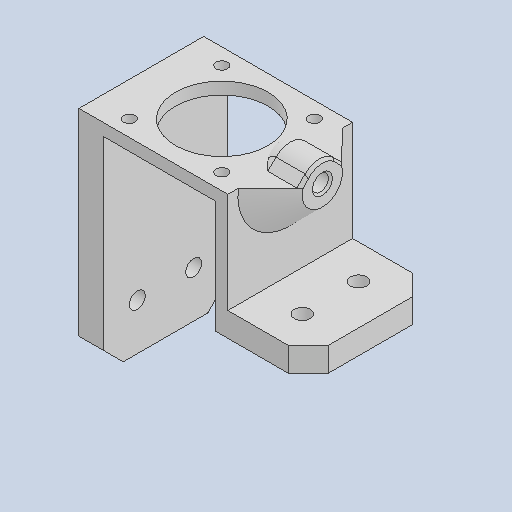
# Autodesk Inventor part: Motor Mount
Saved by Autodesk Inventor 2022 (Build 260153000, 153)
## iProperties
Created: 2022-04-23
Part Number: Motor Mount
Material: Generic
Document SubType Name: Modeling
Designer: Nick
Density: 1 g/cm^3
Appearance: Default
Author: Nick
Autodesk Inventor part; units mm, degrees
ref_plane "YZ Plane" through (0, 0, 0) normal (1, 0, 0) x (0, 1, 0)
ref_plane "XZ Plane" through (0, 0, 0) normal (0, 1, 0) x (-1, 0, 0)
ref_plane "XY Plane" through (0, 0, 0) normal (0, 0, 1) x (1, 0, 0)
sketch "Sketch1" plane through (0, 0, 0) normal (0, 0, 1) x (1, 0, 0)
  line L0 (0, 0) -> (0, 54.05)
  line L1 (0, 54.05) -> (37, 54.05)
  line L2 (37, 54.05) -> (37, 29.05)
  line L3 (37, 29.05) -> (57, 29.05)
  line L4 (57, 29.05) -> (57, 23.05)
  line L5 (57, 23.05) -> (34, 23.05)
  line L6 (34, 23.05) -> (34, 51.05)
  line L7 (34, 51.05) -> (6, 51.05)
  line L8 (6, 51.05) -> (6, 0)
  line L9 (6, 0) -> (0, 0)
  dimension "d0" = 6
  dimension "d1" = 3
  dimension "d2" = 3
  dimension "d3" = 28
  dimension "d5" = 6
  dimension "d6" = 28
  dimension "d7" = 20
  dimension "d60" = 23.05
  constraints: 20 end point, 6 perpendicular, 3 vertical, 1 parallel
  measures "d0" distance of L8.end L0.start
  measures "d1" distance between parallel lines of L1 L7
  measures "d2" distance between parallel lines of L2 L6
  measures "d3" distance of L6.end L7.end
  measures "d5" distance of L3.end L4.end
  measures "d6" distance of L5.end L6.end
  measures "d7" distance of L2.end L3.end
  measures "d60" distance between parallel lines of L9 L5
extrude "Extrusion1" add sketch "Sketch1" along normal blind 31
sketch "Sketch2" plane through (0, 54.05, 0) normal (0, 1, 0) x (1, 0, 0)
  line L0 (8.5, -27) -> (31.5, -27) construction
  line L1 (31.5, -27) -> (31.5, -4) construction
  line L2 (31.5, -4) -> (8.5, -4) construction
  line L3 (8.5, -4) -> (8.5, -27) construction
  line L4 (0, 0) -> (0, -31) construction
  line L5 (37, 0) -> (0, 0) construction
  line L6 (6, 0) -> (34, 0) projected
  line L7 (34, 0) -> (34, -31) projected
  line L8 (6, -31) -> (34, -31) projected
  line L9 (6, 0) -> (6, -31) projected
  point P0 (20, -15.5)
  point P1 (8.5, -15.5)
  point P2 (20, -4)
  point P3 (0, -15.5)
  point P4 (20, 0)
  dimension "d10" = 23
  constraints: 8 end point, 4 midpoint, 2 coincident, 2 horizontal alignment, 2 parallel, 2 perpendicular, 2 vertical alignment, 1 horizontal
  measures "d10" distance of L2.end L0.start
hole "Hole1" at (8.5, 54.05, 27) at (8.5, 54.05, 4) at (31.5, 54.05, 4) at (31.5, 54.05, 27) direction (0, -1, 0) diameter 2.9 end through all
hole "Hole2" at (20, 54.05, 15.5) direction (0, -1, 0) diameter 23 end through all
sketch "Sketch3" plane through (37, 29.05, 0) normal (1, 0, 0) x (0, 0, -1)
  circle A0 centre (-15.5, 23.5) radius 2
  line L0 (0, -6) -> (-31, -6) projected
  circle A1 centre (-15.5, 23.5) radius 5
  point P0 (0, -29.05)
  point P1 (-15.5, -6)
  dimension "d25" = 29.5
  dimension "d26" = 4
  dimension "d27" = 3
  constraints: 2 centre point, 1 midpoint, 1 vertical alignment
  measures "d25" distance from line of A0.centre L0
  measures "d26" diameter of A0
  measures "d27" radial gap between concentric circles of A0 A1
extrude "Extrusion2" add sketch "Sketch3" along normal blind 8
chamfer "Chamfer1" distance 8 angle 45 2 edges at (37, 53.3088, 10.5579) (37, 47.6079, 16.2588)
chamfer "Chamfer2" distance 0.5 angle 45 1 edges at (45, 52.55, 17.5)
sketch "Sketch7" plane through (37, 29.05, 0) normal (0, 1, 0) x (1, 0, 0)
  line L0 (20, 0) -> (0, 0) projected
  line L1 (0, 0) -> (0, -31) projected
  line L2 (20, -31) -> (0, -31) projected
  line L3 (20, 0) -> (20, -31) projected
  point P0 (-37, 0)
  point P1 (10, -22.5)
  point P2 (10, -8.5)
  point P3 (10, -31)
  dimension "d61" = 14
  dimension "d62" = 8.5
  dimension "d63" = 8.5
  constraints: 2 vertical alignment, 1 midpoint
  measures "d61" distance of point (10, -22.5) point (10, -8.5)
  measures "d62" distance of point (10, -31) point (10, -22.5)
  measures "d63" distance from line of L0 point (10, -8.5)
hole "Hole5" at (47, 29.05, 22.5) at (47, 29.05, 8.5) direction (0, -1, 0) diameter 4 end through all
sketch "Sketch8" plane through (0, 0, 0) normal (-1, 0, 0) x (0, 0, 1)
  line L0 (0, 54.05) -> (0, 0) projected
  line L1 (31, 54.05) -> (31, 0) projected
  line L2 (0, 0) -> (31, 0) projected
  line L3 (0, 0) -> (31, 0) construction
  line L4 (31, 0) -> (31, 51.05) construction
  line L5 (0, 0) -> (31, 0) construction
  line L6 (31, 0) -> (31, 23.05) construction
  line L7 (31, 23.05) -> (0, 23.05) construction
  line L8 (0, 23.05) -> (0, 0) construction
  point P0 (8.5, 11.525)
  point P1 (22.5, 11.525)
  point P2 (0, 11.525)
  dimension "d71" = 14
  dimension "d72" = 8.5
  dimension "d73" = 8.5
  dimension "d75" = 23.05
  constraints: 8 end point, 2 horizontal alignment, 2 parallel, 1 horizontal, 1 midpoint, 1 perpendicular, 1 point on line
  measures "d71" distance of point (22.5, 11.525) point (8.5, 11.525)
  measures "d72" distance from line of L0 point (8.5, 11.525)
  measures "d73" distance from line of L1 point (22.5, 11.525)
  measures "d75" distance of L6.end L5.end
hole "Hole6" at (0, 11.525, 8.5) at (0, 11.525, 22.5) direction (1, 0, 0) diameter 4 end through all
chamfer "Chamfer3" distance 5 angle 45 4 edges at (3, 0, 0) (3, 0, 31) (57, 26.05, 31) (57, 26.05, 0)
sketch "Sketch9" plane through (45, 29.05, 0) normal (1, 0, 0) x (0, 0, -1)
  arc A0 (-20.2697, 25) -> (-10.7303, 25) centre (-15.5, 23.5) ccw projected
  arc A1 (-10.7303, 25) -> (-20.2697, 25) centre (-15.5, 23.5) ccw projected
  circle A2 centre (-15.5, 23.5) radius 2.5 projected
  arc A3 (-10.7303, 25) -> (-20.2697, 25) centre (-15.5, 23.5) ccw projected
  line L0 (-11.9645, 27.0355) -> (-9.9289, 25)
  line L1 (-19.0355, 27.0355) -> (-21.0711, 25)
  line L2 (-20.2697, 25) -> (-28.4132, 25) projected
  line L3 (-2.5868, 25) -> (-10.7303, 25) projected
  point P0 (0, -29.05)
  point P1 (-11.9645, 27.0355)
  point P2 (-19.0355, 27.0355)
  dimension "d86" = 45
  constraints: 4 end point, 3 tangent, 2 point on circle, 2 point on line, 1 perpendicular
  measures "d86" angle of L3 L0
extrude "Extrusion3" add sketch "Sketch9" against normal blind 8 contours L2 L1 A1 | A1 L0 L3
sketch "Sketch10" plane through (45, 54.05, 9.9289) normal (0, -1, 0) x (1, 0, 0)
  spline S0 degree 2 poles (0, 0.8014) (-0.3549, 0.4293) (-0.7695, 0) knots 0 0 0 1 1 1 weights 1 1.00278 1 projected
  line L0 (0, 0) -> (-0.7695, 0) projected
  line L1 (0, 0.8014) -> (0, 0) projected
  line L2 (0, 11.1421) -> (0, 10.3408) projected
  line L3 (0, 11.1421) -> (-0.7695, 11.1421) projected
  line L4 (-56.4, 5.5711) -> (23.4, 5.5711) projected
  point P0 (-45, -9.9289)
  constraints: 2 other
sketch3d "3D Sketch1"
  line L0 (45, 54.05, 9.9289) -> (45, 56.0855, 11.9645)
  arc A0 (45, 56.0855, 11.9645) -> (45, 56.0855, 19.0355) centre (45, 52.55, 15.5) ccw
  line L1 (45, 56.0855, 19.0355) -> (45, 54.05, 21.0711)
sweep "Sweep1" cut profiles "Sketch10" path "3D Sketch1"
sketch "Sketch11" plane through (37, 29.05, 0) normal (-1, 0, 0) x (0, 0, 1)
  line L0 (16.8229, 25) -> (21.0711, 25) projected
  line L1 (21.0711, 25) -> (19.0355, 27.0355) projected
  arc A0 (19.0355, 27.0355) -> (11.9645, 27.0355) centre (15.5, 23.5) ccw projected
  line L2 (11.9645, 27.0355) -> (9.9289, 25) projected
  line L3 (9.9289, 25) -> (14.1771, 25) projected
  arc A1 (16.8229, 25) -> (14.1771, 25) centre (15.5, 23.5) ccw projected
  point P0 (0, -29.05)
revolve "Revolution3" add sketch "Sketch11" angle 90 about axis through (37, 54.05, 16.8229) along (0, 0, 1)
equation "\"d6\" = MotorHeight"
equation "\"d62\" = d63"
equation "\"d72\" = d73"
equation "\"MotorHeight\" = MotorHeightBase"
equation "\"MotorHeightBase\" = 28"
body "Solid1"
